Autodesk Inventor part; units mm, degrees
(part 2 of 2)
chamfer "面取り9" distance 1 angle 45 2 edges at (-21.2643, -13.5, -0.5) (21.2643, -13.5, -0.5)
extrude "押し出し12" add sketch "スケッチ5" against normal blind 1 contours L286 L287 L272 L308 L311 A37 | A37 L311 A36 L272 | A36 L311 L272 | A37 L272 A36 L311 | L311 L308 L272 L258 L248 A37 | L311 A36 L272 | L248 L258 L272 | L289 L288 L274 A39 L323 L320 | L320 L323 A39 L274 L262 L261 | L261 L262 L274 | L323 A38 L274 A39 | A39 L274 A38 L323 | L323 L274 A38 | A38 L274 L323 picked at (-26.6892, 18.0876) picked at (-26.0036, 18.1374) picked at (-25.665, 19.7511) picked at (-25.7928, 19.0112) picked at (25.665, 19.7511) picked at (26.7527, 18.6175) picked at (25.7928, 19.0112) picked at (25.9773, 18.9003)
chamfer "面取り10" distance 2 angle 45 2 edges at (-28, 8.5, -0.5) (28, 8.5, -0.5)
chamfer "面取り11" distance 0.8 angle 45 2 edges at (-28, -8.5, -0.5) (28, -8.5, -0.5)
extrude "押し出し13" cut sketch "スケッチ5" against normal blind 1.5 contours A19 | A22 | A25 | A28
extrude "押し出し14" cut sketch "スケッチ5" against normal blind 1.5 contours A30 | A33
extrude "押し出し15" cut sketch "スケッチ5" against normal blind 1.5 contours L314 L260 L275 L295 L310 | L310 L295 L315 L314 | L313 L275 L308 | L308 L275 L258 L314 L313 | L310 L297 L296 L295 | L295 L277 L309 L297 L310 | L314 L258 L275 L260 | L277 L297 L309
chamfer "面取り12" distance 2 angle 45 1 edges at (-23, 13.5, -0.5)
extrude "押し出し16" cut sketch "スケッチ5" against normal blind 1.5 contours L277 L321 L300 | L320 L276 L316 | L316 L317 L261 L276 L320 | L277 L298 L322 L300 L321 | L317 L263 L276 L261 | L276 L263 L317 L322 L298 | L322 L298 L299 L300 | L322 L317 L318 L298
chamfer "面取り13" distance 2 angle 45 1 edges at (23, 13.5, -0.5)
extrude "押し出し17" cut sketch "スケッチ5" against normal blind 1.5 contours A36 L311 L272 | L272 L311 A36 | L311 A36 L272 | L272 A36 L311
extrude "押し出し18" cut sketch "スケッチ5" against normal blind 1.5 contours L323 L274 A38 | A38 L274 L323 | A38 L323 L274 | L274 L323 A38
extrude "押し出し20" cut sketch "スケッチ5" against normal blind 1.5 contours L290 L291 L292 L238
fillet "フィレット1" radius 0.8 4 edges at (-16, 8.5, -0.5) (-16, -8.5, -0.5) (16, -8.5, -0.5) (16, 8.5, -0.5)
fillet "フィレット2" radius 0.8 12 edges at (-23, 15.5, -0.5) (-21, 13.5, -0.5) (-17.8255, 13.5, -0.5) (17.8255, 13.5, -0.5) (21, 13.5, -0.5) (23, 15.5, -0.5) (23, 24.1685, -0.5) (-23, 24.1685, -0.5) (-20.2643, -13.5, -0.5) (-18.2643, -13.5, -0.5) (18.2643, -13.5, -0.5) (20.2643, -13.5, -0.5)
fillet "フィレット3" radius 0.8 24 edges at (-3.6203, -29.5, -0.5) (-5.1203, -31, -0.5) (-9.1203, -31, -0.5) (3.6203, -29.5, -0.5) (5.1203, -31, -0.5) (9.1203, -31, -0.5) (28, -12.5, -0.5) (28, -9.3, -0.5) (27.2, -8.5, -0.5) (26, 8.5, -0.5) (28, 10.5, -0.5) (28, 26.5, -0.5) (23.3435, 30.4073, -0.5) (22.1166, 36.1792, -0.5) (8.558, 47.5563, -0.5) (-8.558, 47.5563, -0.5) (-22.1166, 36.1792, -0.5) (-23.3435, 30.4073, -0.5) (-28, 26.5, -0.5) (-28, 10.5, -0.5) (-26, 8.5, -0.5) (-27.2, -8.5, -0.5) (-28, -9.3, -0.5) (-28, -12.5, -0.5)
extrude "押し出し21" cut sketch "スケッチ5" against normal blind 2 contours L326 L327 L328 L329 | L335 L334 L333 L332 | A41 | A42
